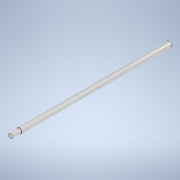
# Autodesk Inventor part: tija filet
Saved by Autodesk Inventor 2021.2 (Build 252289000, 289)
## iProperties
Created: 2024-04-21
Part Number: tija filet
Material: Aluminum 6061-AHC
Document SubType Name: Modeling
Designer: cioba
Density: 2.7 g/cm^3
Appearance: Aluminum - Dark
Author: cioba
Autodesk Inventor part; units mm, degrees
ref_plane "YZ Plane" through (0, 0, 0) normal (1, 0, 0) x (0, 1, 0)
ref_plane "XZ Plane" through (0, 0, 0) normal (0, 1, 0) x (-1, 0, 0)
ref_plane "XY Plane" through (0, 0, 0) normal (0, 0, 1) x (1, 0, 0)
sketch "Sketch1" plane through (0, 0, 0) normal (0, 0, 1) x (1, 0, 0)
  circle A0 centre (-484.1136, 205.0223) radius 3
  circle A1 centre (-484.1136, 205.0223) radius 2.5
  point P0 (0, 0)
  constraints: 2 centre point, 1 coincident
extrude "Extrusion1" add sketch "Sketch1" against normal blind 180 contours A0 | A1
extrude "Extrusion2" cut sketch "Sketch1" against normal blind 10
body "Solid1"
